Autodesk Inventor part; units mm, degrees
(part 2 of 3)
sketch "Эскиз2" plane through (0, 0, 5) normal (0, 0, 1) x (1, 0, 0)
  circle A0 centre (9.1909, 9.1909) radius 1.6
  line L0 (7.3241, 8.9171) -> (8.619, 7.3929)
  line L1 (8.619, 7.3929) -> (11.0578, 9.4648)
  line L2 (11.0578, 9.4648) -> (9.7628, 10.989)
  line L3 (9.7628, 10.989) -> (7.3241, 8.9171)
  line L4 (7.3241, 8.9171) -> (11.0578, 9.4648) construction
  line L5 (8.619, 7.3929) -> (9.7628, 10.989) construction
  line L6 (7.2492, 10.7043) -> (8.0113, 11.3517)
  line L7 (8.0113, 11.3517) -> (8.9245, 10.2768)
  line L8 (8.9245, 10.2768) -> (8.1624, 9.6293)
  line L9 (8.1624, 9.6293) -> (7.2492, 10.7043)
  circle A1 centre (9.1909, 9.1909) radius 0.5
  line L10 (8.5848, 2.046) -> (8.6119, 2.08)
  line L11 (8.6119, 2.08) -> (8.6454, 2.1135)
  line L12 (8.6454, 2.1135) -> (8.6907, 2.1463)
  line L13 (8.6907, 2.1463) -> (8.8034, 2.1753)
  line L14 (8.8034, 2.1753) -> (9.3579, 2.1666)
  line L15 (9.3579, 2.1666) -> (9.4696, 2.1341)
  line L16 (9.4696, 2.1341) -> (9.5139, 2.0998)
  line L17 (9.5139, 2.0998) -> (9.5464, 2.0653)
  line L18 (9.5464, 2.0653) -> (9.5724, 2.0305)
  line L19 (9.5724, 2.0305) -> (9.5941, 1.9955)
  line L20 (9.5941, 1.9955) -> (9.6287, 1.9253)
  line L21 (9.6287, 1.9253) -> (9.6547, 1.8546)
  line L22 (9.6547, 1.8546) -> (9.6746, 1.7836)
  line L23 (9.6746, 1.7836) -> (9.6894, 1.7122)
  line L24 (9.6894, 1.7122) -> (9.7076, 1.5688)
  line L25 (9.7076, 1.5688) -> (9.7394, 1.4264)
  line L26 (9.7394, 1.4264) -> (9.7859, 1.2851)
  line L27 (9.7859, 1.2851) -> (9.8431, 1.1448)
  line L28 (9.8431, 1.1448) -> (9.9095, 1.0056)
  line L29 (9.9095, 1.0056) -> (9.9841, 0.8675)
  line L30 (9.9841, 0.8675) -> (10.0665, 0.7307)
  line L31 (10.0665, 0.7307) -> (10.1561, 0.5952)
  line L32 (10.1561, 0.5952) -> (10.2527, 0.4612)
  line L33 (10.2527, 0.4612) -> (10.356, 0.3288)
  line L34 (10.356, 0.3288) -> (10.4658, 0.1981)
  line L35 (10.4658, 0.1981) -> (10.5522, 0.1014)
  line L36 (10.5522, 0.1014) -> (11.1304, 0.207)
  line L37 (11.1304, 0.207) -> (11.1771, 0.3281)
  line L38 (11.1771, 0.3281) -> (11.2336, 0.4891)
  line L39 (11.2336, 0.4891) -> (11.2834, 0.6494)
  line L40 (11.2834, 0.6494) -> (11.3264, 0.8089)
  line L41 (11.3264, 0.8089) -> (11.3624, 0.9673)
  line L42 (11.3624, 0.9673) -> (11.3911, 1.1244)
  line L43 (11.3911, 1.1244) -> (11.4121, 1.28)
  line L44 (11.4121, 1.28) -> (11.425, 1.4337)
  line L45 (11.425, 1.4337) -> (11.4289, 1.5851)
  line L46 (11.4289, 1.5851) -> (11.4224, 1.7338)
  line L47 (11.4224, 1.7338) -> (11.4018, 1.8782)
  line L48 (11.4018, 1.8782) -> (11.3682, 2.0188)
  line L49 (11.3682, 2.0188) -> (11.3568, 2.0908)
  line L50 (11.3568, 2.0908) -> (11.3503, 2.1643)
  line L51 (11.3503, 2.1643) -> (11.3497, 2.2396)
  line L52 (11.3497, 2.2396) -> (11.3572, 2.3175)
  line L53 (11.3572, 2.3175) -> (11.3651, 2.3579)
  line L54 (11.3651, 2.3579) -> (11.3772, 2.3996)
  line L55 (11.3772, 2.3996) -> (11.3953, 2.4434)
  line L56 (11.3953, 2.4434) -> (11.4247, 2.4911)
  line L57 (11.4247, 2.4911) -> (11.5177, 2.5611)
  line L58 (11.5177, 2.5611) -> (12.0333, 2.7652)
  line L59 (12.0333, 2.7652) -> (12.149, 2.7779)
  line L60 (12.149, 2.7779) -> (12.203, 2.7632)
  line L61 (12.203, 2.7632) -> (12.2462, 2.7437)
  line L62 (12.2462, 2.7437) -> (12.2835, 2.7215)
  line L63 (12.2835, 2.7215) -> (12.317, 2.6976)
  line L64 (12.317, 2.6976) -> (12.3758, 2.6459)
  line L65 (12.3758, 2.6459) -> (12.4269, 2.5905)
  line L66 (12.4269, 2.5905) -> (12.4724, 2.5325)
  line L67 (12.4724, 2.5325) -> (12.5134, 2.4723)
  line L68 (12.5134, 2.4723) -> (12.5852, 2.3468)
  line L69 (12.5852, 2.3468) -> (12.669, 2.2273)
  line L70 (12.669, 2.2273) -> (12.766, 2.1145)
  line L71 (12.766, 2.1145) -> (12.8726, 2.0068)
  line L72 (12.8726, 2.0068) -> (12.9872, 1.9036)
  line L73 (12.9872, 1.9036) -> (13.109, 1.8046)
  line L74 (13.109, 1.8046) -> (13.2375, 1.7097)
  line L75 (13.2375, 1.7097) -> (13.3721, 1.6189)
  line L76 (13.3721, 1.6189) -> (13.5126, 1.532)
  line L77 (13.5126, 1.532) -> (13.6587, 1.4492)
  line L78 (13.6587, 1.4492) -> (13.8101, 1.3705)
  line L79 (13.8101, 1.3705) -> (13.927, 1.3142)
  line L80 (13.927, 1.3142) -> (14.4208, 1.6331)
  line L81 (14.4208, 1.6331) -> (14.4176, 1.7628)
  line L82 (14.4176, 1.7628) -> (14.4082, 1.9332)
  line L83 (14.4082, 1.9332) -> (14.3928, 2.1004)
  line L84 (14.3928, 2.1004) -> (14.3715, 2.2642)
  line L85 (14.3715, 2.2642) -> (14.3441, 2.4243)
  line L86 (14.3441, 2.4243) -> (14.3105, 2.5804)
  line L87 (14.3105, 2.5804) -> (14.2704, 2.7322)
  line L88 (14.2704, 2.7322) -> (14.2235, 2.8791)
  line L89 (14.2235, 2.8791) -> (14.1692, 3.0205)
  line L90 (14.1692, 3.0205) -> (14.1063, 3.1554)
  line L91 (14.1063, 3.1554) -> (14.032, 3.2809)
  line L92 (14.032, 3.2809) -> (13.9471, 3.398)
  line L93 (13.9471, 3.398) -> (13.9091, 3.4601)
  line L94 (13.9091, 3.4601) -> (13.8749, 3.5255)
  line L95 (13.8749, 3.5255) -> (13.8455, 3.5949)
  line L96 (13.8455, 3.5949) -> (13.8226, 3.6697)
  line L97 (13.8226, 3.6697) -> (13.8145, 3.7101)
  line L98 (13.8145, 3.7101) -> (13.8097, 3.7533)
  line L99 (13.8097, 3.7533) -> (13.8097, 3.8007)
  line L100 (13.8097, 3.8007) -> (13.8185, 3.8559)
  line L101 (13.8185, 3.8559) -> (13.8777, 3.9562)
  line L102 (13.8777, 3.9562) -> (14.2759, 4.3421)
  line L103 (14.2759, 4.3421) -> (14.378, 4.398)
  line L104 (14.378, 4.398) -> (14.4335, 4.4051)
  line L105 (14.4335, 4.4051) -> (14.4809, 4.4036)
  line L106 (14.4809, 4.4036) -> (14.5238, 4.3975)
  line L107 (14.5238, 4.3975) -> (14.5639, 4.3881)
  line L108 (14.5639, 4.3881) -> (14.638, 4.3629)
  line L109 (14.638, 4.3629) -> (14.7065, 4.3313)
  line L110 (14.7065, 4.3313) -> (14.7707, 4.2951)
  line L111 (14.7707, 4.2951) -> (14.8316, 4.2551)
  line L112 (14.8316, 4.2551) -> (14.946, 4.1667)
  line L113 (14.946, 4.1667) -> (15.0691, 4.0884)
  line L114 (15.0691, 4.0884) -> (15.2019, 4.0213)
  line L115 (15.2019, 4.0213) -> (15.3416, 3.9626)
  line L116 (15.3416, 3.9626) -> (15.4869, 3.9111)
  line L117 (15.4869, 3.9111) -> (15.6374, 3.8662)
  line L118 (15.6374, 3.8662) -> (15.7924, 3.8277)
  line L119 (15.7924, 3.8277) -> (15.9515, 3.7953)
  line L120 (15.9515, 3.7953) -> (16.1146, 3.7689)
  line L121 (16.1146, 3.7689) -> (16.2812, 3.7483)
  line L122 (16.2812, 3.7483) -> (16.4512, 3.7335)
  line L123 (16.4512, 3.7335) -> (16.5808, 3.7262)
  line L124 (16.5808, 3.7262) -> (16.915, 4.2097)
  line L125 (16.915, 4.2097) -> (16.8624, 4.3284)
  line L126 (16.8624, 4.3284) -> (16.7885, 4.4822)
  line L127 (16.7885, 4.4822) -> (16.7103, 4.6308)
  line L128 (16.7103, 4.6308) -> (16.6279, 4.774)
  line L129 (16.6279, 4.774) -> (16.5413, 4.9114)
  line L130 (16.5413, 4.9114) -> (16.4505, 5.0428)
  line L131 (16.4505, 5.0428) -> (16.3554, 5.1677)
  line L132 (16.3554, 5.1677) -> (16.2558, 5.2855)
  line L133 (16.2558, 5.2855) -> (16.1515, 5.3953)
  line L134 (16.1515, 5.3953) -> (16.0419, 5.4958)
  line L135 (16.0419, 5.4958) -> (15.9251, 5.5834)
  line L136 (15.9251, 5.5834) -> (15.8019, 5.6591)
  line L137 (15.8019, 5.6591) -> (15.743, 5.7019)
  line L138 (15.743, 5.7019) -> (15.6864, 5.7492)
  line L139 (15.6864, 5.7492) -> (15.6327, 5.8021)
  line L140 (15.6327, 5.8021) -> (15.5829, 5.8625)
  line L141 (15.5829, 5.8625) -> (15.56, 5.8967)
  line L142 (15.56, 5.8967) -> (15.539, 5.9347)
  line L143 (15.539, 5.9347) -> (15.5209, 5.9785)
  line L144 (15.5209, 5.9785) -> (15.5079, 6.0329)
  line L145 (15.5079, 6.0329) -> (15.5242, 6.1482)
  line L146 (15.5242, 6.1482) -> (15.7444, 6.6571)
  line L147 (15.7444, 6.6571) -> (15.8173, 6.7479)
  line L148 (15.8173, 6.7479) -> (15.8658, 6.7757)
  line L149 (15.8658, 6.7757) -> (15.9102, 6.7924)
  line L150 (15.9102, 6.7924) -> (15.9523, 6.8032)
  line L151 (15.9523, 6.8032) -> (15.9929, 6.8099)
  line L152 (15.9929, 6.8099) -> (16.071, 6.8149)
  line L153 (16.071, 6.8149) -> (16.1463, 6.812)
  line L154 (16.1463, 6.812) -> (16.2195, 6.8031)
  line L155 (16.2195, 6.8031) -> (16.2911, 6.7895)
  line L156 (16.2911, 6.7895) -> (16.4306, 6.7515)
  line L157 (16.4306, 6.7515) -> (16.5743, 6.7263)
  line L158 (16.5743, 6.7263) -> (16.7227, 6.7151)
  line L159 (16.7227, 6.7151) -> (16.8742, 6.7143)
  line L160 (16.8742, 6.7143) -> (17.0282, 6.7224)
  line L161 (17.0282, 6.7224) -> (17.1843, 6.7385)
  line L162 (17.1843, 6.7385) -> (17.3423, 6.7622)
  line L163 (17.3423, 6.7622) -> (17.5017, 6.7932)
  line L164 (17.5017, 6.7932) -> (17.6625, 6.8312)
  line L165 (17.6625, 6.8312) -> (17.8243, 6.8759)
  line L166 (17.8243, 6.8759) -> (17.987, 6.9273)
  line L167 (17.987, 6.9273) -> (18.1095, 6.9702)
  line L168 (18.1095, 6.9702) -> (18.2332, 7.5448)
  line L169 (18.2332, 7.5448) -> (18.1392, 7.6343)
  line L170 (18.1392, 7.6343) -> (18.0121, 7.7481)
  line L171 (18.0121, 7.7481) -> (17.883, 7.8555)
  line L172 (17.883, 7.8555) -> (17.7521, 7.9562)
  line L173 (17.7521, 7.9562) -> (17.6195, 8.0501)
  line L174 (17.6195, 8.0501) -> (17.4854, 8.1367)
  line L175 (17.4854, 8.1367) -> (17.3497, 8.2156)
  line L176 (17.3497, 8.2156) -> (17.2126, 8.2864)
  line L177 (17.2126, 8.2864) -> (17.0742, 8.348)
  line L178 (17.0742, 8.348) -> (16.9344, 8.3988)
  line L179 (16.9344, 8.3988) -> (16.7931, 8.4351)
  line L180 (16.7931, 8.4351) -> (16.6503, 8.4578)
  line L181 (16.6503, 8.4578) -> (16.5795, 8.4749)
  line L182 (16.5795, 8.4749) -> (16.5091, 8.4969)
  line L183 (16.5091, 8.4969) -> (16.4393, 8.5252)
  line L184 (16.4393, 8.5252) -> (16.3701, 8.5619)
  line L185 (16.3701, 8.5619) -> (16.3359, 8.5848)
  line L186 (16.3359, 8.5848) -> (16.3019, 8.6119)
  line L187 (16.3019, 8.6119) -> (16.2684, 8.6454)
  line L188 (16.2684, 8.6454) -> (16.2356, 8.6907)
  line L189 (16.2356, 8.6907) -> (16.2065, 8.8034)
  line L190 (16.2065, 8.8034) -> (16.2152, 9.3579)
  line L191 (16.2152, 9.3579) -> (16.2478, 9.4696)
  line L192 (16.2478, 9.4696) -> (16.282, 9.5139)
  line L193 (16.282, 9.5139) -> (16.3166, 9.5464)
  line L194 (16.3166, 9.5464) -> (16.3514, 9.5724)
  line L195 (16.3514, 9.5724) -> (16.3863, 9.5941)
  line L196 (16.3863, 9.5941) -> (16.4566, 9.6287)
  line L197 (16.4566, 9.6287) -> (16.5273, 9.6547)
  line L198 (16.5273, 9.6547) -> (16.5983, 9.6746)
  line L199 (16.5983, 9.6746) -> (16.6696, 9.6894)
  line L200 (16.6696, 9.6894) -> (16.813, 9.7076)
  line L201 (16.813, 9.7076) -> (16.9555, 9.7394)
  line L202 (16.9555, 9.7394) -> (17.0968, 9.7859)
  line L203 (17.0968, 9.7859) -> (17.2371, 9.8431)
  line L204 (17.2371, 9.8431) -> (17.3763, 9.9095)
  line L205 (17.3763, 9.9095) -> (17.5144, 9.9841)
  line L206 (17.5144, 9.9841) -> (17.6512, 10.0665)
  line L207 (17.6512, 10.0665) -> (17.7867, 10.1561)
  line L208 (17.7867, 10.1561) -> (17.9207, 10.2527)
  line L209 (17.9207, 10.2527) -> (18.0531, 10.356)
  line L210 (18.0531, 10.356) -> (18.1837, 10.4658)
  line L211 (18.1837, 10.4658) -> (18.2805, 10.5522)
  line L212 (18.2805, 10.5522) -> (18.1749, 11.1304)
  line L213 (18.1749, 11.1304) -> (18.0538, 11.1771)
  line L214 (18.0538, 11.1771) -> (17.8928, 11.2336)
  line L215 (17.8928, 11.2336) -> (17.7324, 11.2834)
  line L216 (17.7324, 11.2834) -> (17.5729, 11.3264)
  line L217 (17.5729, 11.3264) -> (17.4145, 11.3624)
  line L218 (17.4145, 11.3624) -> (17.2574, 11.3911)
  line L219 (17.2574, 11.3911) -> (17.1019, 11.4121)
  line L220 (17.1019, 11.4121) -> (16.9482, 11.425)
  line L221 (16.9482, 11.425) -> (16.7967, 11.4289)
  line L222 (16.7967, 11.4289) -> (16.6481, 11.4224)
  line L223 (16.6481, 11.4224) -> (16.5036, 11.4018)
  line L224 (16.5036, 11.4018) -> (16.363, 11.3682)
  line L225 (16.363, 11.3682) -> (16.2911, 11.3568)
  line L226 (16.2911, 11.3568) -> (16.2176, 11.3503)
  line L227 (16.2176, 11.3503) -> (16.1423, 11.3497)
  line L228 (16.1423, 11.3497) -> (16.0643, 11.3572)
  line L229 (16.0643, 11.3572) -> (16.0239, 11.3651)
  line L230 (16.0239, 11.3651) -> (15.9822, 11.3772)
  line L231 (15.9822, 11.3772) -> (15.9384, 11.3953)
  line L232 (15.9384, 11.3953) -> (15.8907, 11.4247)
  line L233 (15.8907, 11.4247) -> (15.8208, 11.5177)
  line L234 (15.8208, 11.5177) -> (15.6166, 12.0333)
  line L235 (15.6166, 12.0333) -> (15.604, 12.149)
  line L236 (15.604, 12.149) -> (15.6187, 12.203)
  line L237 (15.6187, 12.203) -> (15.6382, 12.2462)
  line L238 (15.6382, 12.2462) -> (15.6603, 12.2835)
  line L239 (15.6603, 12.2835) -> (15.6843, 12.317)
  line L240 (15.6843, 12.317) -> (15.736, 12.3758)
  line L241 (15.736, 12.3758) -> (15.7913, 12.4269)
  line L242 (15.7913, 12.4269) -> (15.8494, 12.4724)
  line L243 (15.8494, 12.4724) -> (15.9096, 12.5134)
  line L244 (15.9096, 12.5134) -> (16.0351, 12.5852)
  line L245 (16.0351, 12.5852) -> (16.1546, 12.669)
  line L246 (16.1546, 12.669) -> (16.2673, 12.766)
  line L247 (16.2673, 12.766) -> (16.375, 12.8726)
  line L248 (16.375, 12.8726) -> (16.4783, 12.9872)
  line L249 (16.4783, 12.9872) -> (16.5772, 13.109)
  line L250 (16.5772, 13.109) -> (16.6721, 13.2375)
  line L251 (16.6721, 13.2375) -> (16.763, 13.3721)
  line L252 (16.763, 13.3721) -> (16.8498, 13.5126)
  line L253 (16.8498, 13.5126) -> (16.9326, 13.6587)
  line L254 (16.9326, 13.6587) -> (17.0113, 13.8101)
  line L255 (17.0113, 13.8101) -> (17.0676, 13.927)
  line L256 (17.0676, 13.927) -> (16.7488, 14.4208)
  line L257 (16.7488, 14.4208) -> (16.6191, 14.4176)
  line L258 (16.6191, 14.4176) -> (16.4487, 14.4082)
  line L259 (16.4487, 14.4082) -> (16.2815, 14.3928)
  line L260 (16.2815, 14.3928) -> (16.1177, 14.3715)
  line L261 (16.1177, 14.3715) -> (15.9576, 14.3441)
  line L262 (15.9576, 14.3441) -> (15.8015, 14.3105)
  line L263 (15.8015, 14.3105) -> (15.6497, 14.2704)
  line L264 (15.6497, 14.2704) -> (15.5028, 14.2235)
  line L265 (15.5028, 14.2235) -> (15.3613, 14.1692)
  line L266 (15.3613, 14.1692) -> (15.2265, 14.1063)
  line L267 (15.2265, 14.1063) -> (15.1009, 14.032)
  line L268 (15.1009, 14.032) -> (14.9839, 13.9471)
  line L269 (14.9839, 13.9471) -> (14.9217, 13.9091)
  line L270 (14.9217, 13.9091) -> (14.8564, 13.8749)
  line L271 (14.8564, 13.8749) -> (14.787, 13.8455)
  line L272 (14.787, 13.8455) -> (14.7121, 13.8226)
  line L273 (14.7121, 13.8226) -> (14.6718, 13.8145)
  line L274 (14.6718, 13.8145) -> (14.6286, 13.8097)
  line L275 (14.6286, 13.8097) -> (14.5812, 13.8097)
  line L276 (14.5812, 13.8097) -> (14.5259, 13.8185)
  line L277 (14.5259, 13.8185) -> (14.4257, 13.8777)
  line L278 (14.4257, 13.8777) -> (14.0398, 14.2759)
  line L279 (14.0398, 14.2759) -> (13.9838, 14.378)
  line L280 (13.9838, 14.378) -> (13.9767, 14.4335)
  line L281 (13.9767, 14.4335) -> (13.9782, 14.4809)
  line L282 (13.9782, 14.4809) -> (13.9844, 14.5238)
  line L283 (13.9844, 14.5238) -> (13.9938, 14.5639)
  line L284 (13.9938, 14.5639) -> (14.019, 14.638)
  line L285 (14.019, 14.638) -> (14.0505, 14.7065)
  line L286 (14.0505, 14.7065) -> (14.0868, 14.7707)
  line L287 (14.0868, 14.7707) -> (14.1267, 14.8316)
  line L288 (14.1267, 14.8316) -> (14.2152, 14.946)
  line L289 (14.2152, 14.946) -> (14.2935, 15.0691)
  line L290 (14.2935, 15.0691) -> (14.3605, 15.2019)
  line L291 (14.3605, 15.2019) -> (14.4193, 15.3416)
  line L292 (14.4193, 15.3416) -> (14.4708, 15.4869)
  line L293 (14.4708, 15.4869) -> (14.5156, 15.6374)
  line L294 (14.5156, 15.6374) -> (14.5541, 15.7924)
  line L295 (14.5541, 15.7924) -> (14.5866, 15.9515)
  line L296 (14.5866, 15.9515) -> (14.613, 16.1146)
  line L297 (14.613, 16.1146) -> (14.6336, 16.2812)
  line L298 (14.6336, 16.2812) -> (14.6484, 16.4512)
  line L299 (14.6484, 16.4512) -> (14.6556, 16.5808)
  line L300 (14.6556, 16.5808) -> (14.1721, 16.915)
  line L301 (14.1721, 16.915) -> (14.0535, 16.8624)
  line L302 (14.0535, 16.8624) -> (13.8997, 16.7885)
  line L303 (13.8997, 16.7885) -> (13.7511, 16.7103)
  line L304 (13.7511, 16.7103) -> (13.6079, 16.6279)
  line L305 (13.6079, 16.6279) -> (13.4704, 16.5413)
  line L306 (13.4704, 16.5413) -> (13.3391, 16.4505)
  line L307 (13.3391, 16.4505) -> (13.2142, 16.3554)
  line L308 (13.2142, 16.3554) -> (13.0964, 16.2558)
  line L309 (13.0964, 16.2558) -> (12.9865, 16.1515)
  line L310 (12.9865, 16.1515) -> (12.886, 16.0419)
  line L311 (12.886, 16.0419) -> (12.7985, 15.9251)
  line L312 (12.7985, 15.9251) -> (12.7228, 15.8019)
  line L313 (12.7228, 15.8019) -> (12.6799, 15.743)
  line L314 (12.6799, 15.743) -> (12.6327, 15.6864)
  line L315 (12.6327, 15.6864) -> (12.5798, 15.6327)
  line L316 (12.5798, 15.6327) -> (12.5194, 15.5829)
  line L317 (12.5194, 15.5829) -> (12.4852, 15.56)
  line L318 (12.4852, 15.56) -> (12.4472, 15.539)
  line L319 (12.4472, 15.539) -> (12.4034, 15.5209)
  line L320 (12.4034, 15.5209) -> (12.3489, 15.5079)
  line L321 (12.3489, 15.5079) -> (12.2337, 15.5242)
  line L322 (12.2337, 15.5242) -> (11.7248, 15.7444)
  line L323 (11.7248, 15.7444) -> (11.634, 15.8173)
  line L324 (11.634, 15.8173) -> (11.6062, 15.8658)
  line L325 (11.6062, 15.8658) -> (11.5894, 15.9102)
  line L326 (11.5894, 15.9102) -> (11.5787, 15.9523)
  line L327 (11.5787, 15.9523) -> (11.572, 15.9929)
  line L328 (11.572, 15.9929) -> (11.567, 16.071)
  line L329 (11.567, 16.071) -> (11.5699, 16.1463)
  line L330 (11.5699, 16.1463) -> (11.5788, 16.2195)
  line L331 (11.5788, 16.2195) -> (11.5924, 16.2911)
  line L332 (11.5924, 16.2911) -> (11.6304, 16.4306)
  line L333 (11.6304, 16.4306) -> (11.6556, 16.5743)
  line L334 (11.6556, 16.5743) -> (11.6667, 16.7227)
  line L335 (11.6667, 16.7227) -> (11.6676, 16.8742)
  line L336 (11.6676, 16.8742) -> (11.6595, 17.0282)
  line L337 (11.6595, 17.0282) -> (11.6434, 17.1843)
  line L338 (11.6434, 17.1843) -> (11.6196, 17.3423)
  line L339 (11.6196, 17.3423) -> (11.5887, 17.5017)
  line L340 (11.5887, 17.5017) -> (11.5507, 17.6625)
  line L341 (11.5507, 17.6625) -> (11.506, 17.8243)
  line L342 (11.506, 17.8243) -> (11.4545, 17.987)
  line L343 (11.4545, 17.987) -> (11.4117, 18.1095)
  line L344 (11.4117, 18.1095) -> (10.8371, 18.2332)
  line L345 (10.8371, 18.2332) -> (10.7476, 18.1392)
  line L346 (10.7476, 18.1392) -> (10.6338, 18.0121)
  line L347 (10.6338, 18.0121) -> (10.5264, 17.883)
  line L348 (10.5264, 17.883) -> (10.4256, 17.7521)
  line L349 (10.4256, 17.7521) -> (10.3318, 17.6195)
  line L350 (10.3318, 17.6195) -> (10.2452, 17.4854)
  line L351 (10.2452, 17.4854) -> (10.1662, 17.3497)
  line L352 (10.1662, 17.3497) -> (10.0955, 17.2126)
  line L353 (10.0955, 17.2126) -> (10.0339, 17.0742)
  line L354 (10.0339, 17.0742) -> (9.983, 16.9344)
  line L355 (9.983, 16.9344) -> (9.9468, 16.7931)
  line L356 (9.9468, 16.7931) -> (9.924, 16.6503)
  line L357 (9.924, 16.6503) -> (9.907, 16.5795)
  line L358 (9.907, 16.5795) -> (9.885, 16.5091)
  line L359 (9.885, 16.5091) -> (9.8567, 16.4393)
  line L360 (9.8567, 16.4393) -> (9.8199, 16.3701)
  line L361 (9.8199, 16.3701) -> (9.7971, 16.3359)
  line L362 (9.7971, 16.3359) -> (9.77, 16.3019)
  line L363 (9.77, 16.3019) -> (9.7365, 16.2684)
  line L364 (9.7365, 16.2684) -> (9.6911, 16.2356)
  line L365 (9.6911, 16.2356) -> (9.5784, 16.2065)
  line L366 (9.5784, 16.2065) -> (9.024, 16.2152)
  line L367 (9.024, 16.2152) -> (8.9122, 16.2478)
  line L368 (8.9122, 16.2478) -> (8.868, 16.282)
  line L369 (8.868, 16.282) -> (8.8355, 16.3166)
  line L370 (8.8355, 16.3166) -> (8.8095, 16.3514)
  line L371 (8.8095, 16.3514) -> (8.7878, 16.3863)
  line L372 (8.7878, 16.3863) -> (8.7532, 16.4566)
  line L373 (8.7532, 16.4566) -> (8.7271, 16.5273)
  line L374 (8.7271, 16.5273) -> (8.7073, 16.5983)
  line L375 (8.7073, 16.5983) -> (8.6925, 16.6696)
  line L376 (8.6925, 16.6696) -> (8.6742, 16.813)
  line L377 (8.6742, 16.813) -> (8.6425, 16.9555)
  line L378 (8.6425, 16.9555) -> (8.596, 17.0968)
  line L379 (8.596, 17.0968) -> (8.5388, 17.2371)
  line L380 (8.5388, 17.2371) -> (8.4724, 17.3763)
  line L381 (8.4724, 17.3763) -> (8.3977, 17.5144)
  line L382 (8.3977, 17.5144) -> (8.3154, 17.6512)
  line L383 (8.3154, 17.6512) -> (8.2257, 17.7867)
  line L384 (8.2257, 17.7867) -> (8.1291, 17.9207)
  line L385 (8.1291, 17.9207) -> (8.0259, 18.0531)
  line L386 (8.0259, 18.0531) -> (7.9161, 18.1837)
  line L387 (7.9161, 18.1837) -> (7.8296, 18.2805)
  line L388 (7.8296, 18.2805) -> (7.2514, 18.1749)
  line L389 (7.2514, 18.1749) -> (7.2047, 18.0538)
  line L390 (7.2047, 18.0538) -> (7.1482, 17.8928)
  line L391 (7.1482, 17.8928) -> (7.0984, 17.7324)
  line L392 (7.0984, 17.7324) -> (7.0554, 17.5729)
  line L393 (7.0554, 17.5729) -> (7.0195, 17.4145)
  line L394 (7.0195, 17.4145) -> (6.9908, 17.2574)
  line L395 (6.9908, 17.2574) -> (6.9698, 17.1019)
  line L396 (6.9698, 17.1019) -> (6.9569, 16.9482)
  line L397 (6.9569, 16.9482) -> (6.9529, 16.7967)
  line L398 (6.9529, 16.7967) -> (6.9594, 16.6481)
  line L399 (6.9594, 16.6481) -> (6.9801, 16.5036)
  line L400 (6.9801, 16.5036) -> (7.0137, 16.363)
  line L401 (7.0137, 16.363) -> (7.025, 16.2911)
  line L402 (7.025, 16.2911) -> (7.0316, 16.2176)
  line L403 (7.0316, 16.2176) -> (7.0322, 16.1423)
  line L404 (7.0322, 16.1423) -> (7.0247, 16.0643)
  line L405 (7.0247, 16.0643) -> (7.0167, 16.0239)
  line L406 (7.0167, 16.0239) -> (7.0047, 15.9822)
  line L407 (7.0047, 15.9822) -> (6.9865, 15.9384)
  line L408 (6.9865, 15.9384) -> (6.9572, 15.8907)
  line L409 (6.9572, 15.8907) -> (6.8642, 15.8208)
  line L410 (6.8642, 15.8208) -> (6.3486, 15.6166)
  line L411 (6.3486, 15.6166) -> (6.2329, 15.604)
  line L412 (6.2329, 15.604) -> (6.1789, 15.6187)
  line L413 (6.1789, 15.6187) -> (6.1357, 15.6382)
  line L414 (6.1357, 15.6382) -> (6.0983, 15.6603)
  line L415 (6.0983, 15.6603) -> (6.0649, 15.6843)
  line L416 (6.0649, 15.6843) -> (6.0061, 15.736)
  line L417 (6.0061, 15.736) -> (5.9549, 15.7913)
  line L418 (5.9549, 15.7913) -> (5.9094, 15.8494)
  line L419 (5.9094, 15.8494) -> (5.8685, 15.9096)
  line L420 (5.8685, 15.9096) -> (5.7967, 16.0351)
  line L421 (5.7967, 16.0351) -> (5.7129, 16.1546)
  line L422 (5.7129, 16.1546) -> (5.6158, 16.2673)
  line L423 (5.6158, 16.2673) -> (5.5093, 16.375)
  line L424 (5.5093, 16.375) -> (5.3947, 16.4783)
  line L425 (5.3947, 16.4783) -> (5.2729, 16.5772)
  line L426 (5.2729, 16.5772) -> (5.1444, 16.6721)
  line L427 (5.1444, 16.6721) -> (5.0098, 16.763)
  line L428 (5.0098, 16.763) -> (4.8692, 16.8498)
  line L429 (4.8692, 16.8498) -> (4.7232, 16.9326)
  line L430 (4.7232, 16.9326) -> (4.5717, 17.0113)
  line L431 (4.5717, 17.0113) -> (4.4548, 17.0676)
  line L432 (4.4548, 17.0676) -> (3.961, 16.7488)
  line L433 (3.961, 16.7488) -> (3.9643, 16.6191)
  line L434 (3.9643, 16.6191) -> (3.9737, 16.4487)
  line L435 (3.9737, 16.4487) -> (3.989, 16.2815)
  line L436 (3.989, 16.2815) -> (4.0103, 16.1177)
  line L437 (4.0103, 16.1177) -> (4.0377, 15.9576)
  line L438 (4.0377, 15.9576) -> (4.0714, 15.8015)
  line L439 (4.0714, 15.8015) -> (4.1115, 15.6497)
  line L440 (4.1115, 15.6497) -> (4.1584, 15.5028)
  line L441 (4.1584, 15.5028) -> (4.2127, 15.3613)
  line L442 (4.2127, 15.3613) -> (4.2755, 15.2265)
  line L443 (4.2755, 15.2265) -> (4.3499, 15.1009)
  line L444 (4.3499, 15.1009) -> (4.4348, 14.9839)
  line L445 (4.4348, 14.9839) -> (4.4728, 14.9217)
  line L446 (4.4728, 14.9217) -> (4.507, 14.8564)
  line L447 (4.507, 14.8564) -> (4.5364, 14.787)
  line L448 (4.5364, 14.787) -> (4.5593, 14.7121)
  line L449 (4.5593, 14.7121) -> (4.5673, 14.6718)
  line L450 (4.5673, 14.6718) -> (4.5722, 14.6286)
  line L451 (4.5722, 14.6286) -> (4.5722, 14.5812)
  line L452 (4.5722, 14.5812) -> (4.5633, 14.5259)
  line L453 (4.5633, 14.5259) -> (4.5042, 14.4257)
  line L454 (4.5042, 14.4257) -> (4.106, 14.0398)
  line L455 (4.106, 14.0398) -> (4.0039, 13.9838)
  line L456 (4.0039, 13.9838) -> (3.9484, 13.9767)
  line L457 (3.9484, 13.9767) -> (3.901, 13.9782)
  line L458 (3.901, 13.9782) -> (3.858, 13.9844)
  line L459 (3.858, 13.9844) -> (3.8179, 13.9938)
  line L460 (3.8179, 13.9938) -> (3.7438, 14.019)
  line L461 (3.7438, 14.019) -> (3.6754, 14.0505)
  line L462 (3.6754, 14.0505) -> (3.6112, 14.0868)
  line L463 (3.6112, 14.0868) -> (3.5502, 14.1267)
  line L464 (3.5502, 14.1267) -> (3.4359, 14.2152)
  line L465 (3.4359, 14.2152) -> (3.3127, 14.2935)
  line L466 (3.3127, 14.2935) -> (3.18, 14.3605)
  line L467 (3.18, 14.3605) -> (3.0403, 14.4193)
  line L468 (3.0403, 14.4193) -> (2.8949, 14.4708)
  line L469 (2.8949, 14.4708) -> (2.7445, 14.5156)
  line L470 (2.7445, 14.5156) -> (2.5895, 14.5541)
  line L471 (2.5895, 14.5541) -> (2.4303, 14.5866)
  line L472 (2.4303, 14.5866) -> (2.2673, 14.613)
  line L473 (2.2673, 14.613) -> (2.1006, 14.6336)
  line L474 (2.1006, 14.6336) -> (1.9306, 14.6484)
  line L475 (1.9306, 14.6484) -> (1.8011, 14.6556)
  line L476 (1.8011, 14.6556) -> (1.4669, 14.1721)
  line L477 (1.4669, 14.1721) -> (1.5195, 14.0535)
  line L478 (1.5195, 14.0535) -> (1.5934, 13.8997)
  line L479 (1.5934, 13.8997) -> (1.6716, 13.7511)
  line L480 (1.6716, 13.7511) -> (1.7539, 13.6079)
  line L481 (1.7539, 13.6079) -> (1.8405, 13.4704)
  line L482 (1.8405, 13.4704) -> (1.9313, 13.3391)
  line L483 (1.9313, 13.3391) -> (2.0265, 13.2142)
  line L484 (2.0265, 13.2142) -> (2.126, 13.0964)
  line L485 (2.126, 13.0964) -> (2.2303, 12.9865)
  line L486 (2.2303, 12.9865) -> (2.34, 12.886)
  line L487 (2.34, 12.886) -> (2.4568, 12.7985)
  line L488 (2.4568, 12.7985) -> (2.5799, 12.7228)
  line L489 (2.5799, 12.7228) -> (2.6389, 12.6799)
  line L490 (2.6389, 12.6799) -> (2.6954, 12.6327)
  line L491 (2.6954, 12.6327) -> (2.7491, 12.5798)
  line L492 (2.7491, 12.5798) -> (2.799, 12.5194)
  line L493 (2.799, 12.5194) -> (2.8219, 12.4852)
  line L494 (2.8219, 12.4852) -> (2.8428, 12.4472)
  line L495 (2.8428, 12.4472) -> (2.861, 12.4034)
  line L496 (2.861, 12.4034) -> (2.874, 12.3489)
  line L497 (2.874, 12.3489) -> (2.8577, 12.2337)
  line L498 (2.8577, 12.2337) -> (2.6374, 11.7248)
  line L499 (2.6374, 11.7248) -> (2.5646, 11.634)
  line L500 (2.5646, 11.634) -> (2.516, 11.6062)
  line L501 (2.516, 11.6062) -> (2.4717, 11.5894)
  line L502 (2.4717, 11.5894) -> (2.4296, 11.5787)
  line L503 (2.4296, 11.5787) -> (2.389, 11.572)
  line L504 (2.389, 11.572) -> (2.3108, 11.567)
  line L505 (2.3108, 11.567) -> (2.2356, 11.5699)
  line L506 (2.2356, 11.5699) -> (2.1623, 11.5788)
  line L507 (2.1623, 11.5788) -> (2.0908, 11.5924)
  line L508 (2.0908, 11.5924) -> (1.9513, 11.6304)
  line L509 (1.9513, 11.6304) -> (1.8075, 11.6556)
  line L510 (1.8075, 11.6556) -> (1.6592, 11.6667)
  line L511 (1.6592, 11.6667) -> (1.5077, 11.6676)
  line L512 (1.5077, 11.6676) -> (1.3537, 11.6595)
  line L513 (1.3537, 11.6595) -> (1.1975, 11.6434)
  line L514 (1.1975, 11.6434) -> (1.0396, 11.6196)
  line L515 (1.0396, 11.6196) -> (0.8801, 11.5887)
  line L516 (0.8801, 11.5887) -> (0.7194, 11.5507)
  line L517 (0.7194, 11.5507) -> (0.5575, 11.506)
  line L518 (0.5575, 11.506) -> (0.3948, 11.4545)
  line L519 (0.3948, 11.4545) -> (0.2723, 11.4117)
  line L520 (0.2723, 11.4117) -> (0.1486, 10.8371)
  line L521 (0.1486, 10.8371) -> (0.2426, 10.7476)
  line L522 (0.2426, 10.7476) -> (0.3698, 10.6338)
  line L523 (0.3698, 10.6338) -> (0.4988, 10.5264)
  line L524 (0.4988, 10.5264) -> (0.6297, 10.4256)
  line L525 (0.6297, 10.4256) -> (0.7623, 10.3318)
  line L526 (0.7623, 10.3318) -> (0.8965, 10.2452)
  line L527 (0.8965, 10.2452) -> (1.0322, 10.1662)
  line L528 (1.0322, 10.1662) -> (1.1692, 10.0955)
  line L529 (1.1692, 10.0955) -> (1.3077, 10.0339)
  line L530 (1.3077, 10.0339) -> (1.4474, 9.983)
  line L531 (1.4474, 9.983) -> (1.5888, 9.9468)
  line L532 (1.5888, 9.9468) -> (1.7316, 9.924)
  line L533 (1.7316, 9.924) -> (1.8024, 9.907)
  line L534 (1.8024, 9.907) -> (1.8728, 9.885)
  line L535 (1.8728, 9.885) -> (1.9426, 9.8567)
  line L536 (1.9426, 9.8567) -> (2.0118, 9.8199)
  line L537 (2.0118, 9.8199) -> (2.046, 9.7971)
  line L538 (2.046, 9.7971) -> (2.08, 9.77)
  line L539 (2.08, 9.77) -> (2.1135, 9.7365)
  line L540 (2.1135, 9.7365) -> (2.1463, 9.6911)
  line L541 (2.1463, 9.6911) -> (2.1753, 9.5784)
  line L542 (2.1753, 9.5784) -> (2.1666, 9.024)
  line L543 (2.1666, 9.024) -> (2.1341, 8.9122)
  line L544 (2.1341, 8.9122) -> (2.0998, 8.868)
  line L545 (2.0998, 8.868) -> (2.0653, 8.8355)
  line L546 (2.0653, 8.8355) -> (2.0305, 8.8095)
  line L547 (2.0305, 8.8095) -> (1.9956, 8.7878)
  line L548 (1.9956, 8.7878) -> (1.9253, 8.7532)
  line L549 (1.9253, 8.7532) -> (1.8546, 8.7271)
  line L550 (1.8546, 8.7271) -> (1.7836, 8.7073)
  line L551 (1.7836, 8.7073) -> (1.7122, 8.6925)
  line L552 (1.7122, 8.6925) -> (1.5688, 8.6742)
  line L553 (1.5688, 8.6742) -> (1.4264, 8.6425)
  line L554 (1.4264, 8.6425) -> (1.2851, 8.596)
  line L555 (1.2851, 8.596) -> (1.1448, 8.5388)
  line L556 (1.1448, 8.5388) -> (1.0056, 8.4724)
  line L557 (1.0056, 8.4724) -> (0.8675, 8.3977)
  line L558 (0.8675, 8.3977) -> (0.7307, 8.3154)
  line L559 (0.7307, 8.3154) -> (0.5952, 8.2257)
  line L560 (0.5952, 8.2257) -> (0.4612, 8.1291)
  line L561 (0.4612, 8.1291) -> (0.3288, 8.0259)
  line L562 (0.3288, 8.0259) -> (0.1981, 7.9161)
  line L563 (0.1981, 7.9161) -> (0.1014, 7.8296)
  line L564 (0.1014, 7.8296) -> (0.207, 7.2514)
  line L565 (0.207, 7.2514) -> (0.3281, 7.2047)
  line L566 (0.3281, 7.2047) -> (0.4891, 7.1482)
  line L567 (0.4891, 7.1482) -> (0.6494, 7.0984)
  line L568 (0.6494, 7.0984) -> (0.8089, 7.0554)
  line L569 (0.8089, 7.0554) -> (0.9673, 7.0195)
  line L570 (0.9673, 7.0195) -> (1.1244, 6.9908)
  line L571 (1.1244, 6.9908) -> (1.28, 6.9698)
  line L572 (1.28, 6.9698) -> (1.4337, 6.9569)
  line L573 (1.4337, 6.9569) -> (1.5851, 6.9529)
  line L574 (1.5851, 6.9529) -> (1.7337, 6.9594)
  line L575 (1.7337, 6.9594) -> (1.8782, 6.9801)
  line L576 (1.8782, 6.9801) -> (2.0188, 7.0137)
  line L577 (2.0188, 7.0137) -> (2.0908, 7.025)
  line L578 (2.0908, 7.025) -> (2.1643, 7.0316)
  line L579 (2.1643, 7.0316) -> (2.2396, 7.0322)
  line L580 (2.2396, 7.0322) -> (2.3175, 7.0247)
  line L581 (2.3175, 7.0247) -> (2.3579, 7.0167)
  line L582 (2.3579, 7.0167) -> (2.3996, 7.0047)
  line L583 (2.3996, 7.0047) -> (2.4435, 6.9865)
  line L584 (2.4435, 6.9865) -> (2.4911, 6.9572)
  line L585 (2.4911, 6.9572) -> (2.5611, 6.8642)
  line L586 (2.5611, 6.8642) -> (2.7652, 6.3486)
  line L587 (2.7652, 6.3486) -> (2.7779, 6.2329)
  line L588 (2.7779, 6.2329) -> (2.7632, 6.1789)
  line L589 (2.7632, 6.1789) -> (2.7437, 6.1357)
  line L590 (2.7437, 6.1357) -> (2.7215, 6.0983)
  line L591 (2.7215, 6.0983) -> (2.6976, 6.0649)
  line L592 (2.6976, 6.0649) -> (2.6459, 6.0061)
  line L593 (2.6459, 6.0061) -> (2.5905, 5.9549)
  line L594 (2.5905, 5.9549) -> (2.5325, 5.9094)
  line L595 (2.5325, 5.9094) -> (2.4723, 5.8685)
  line L596 (2.4723, 5.8685) -> (2.3468, 5.7967)
  line L597 (2.3468, 5.7967) -> (2.2273, 5.7129)
  line L598 (2.2273, 5.7129) -> (2.1145, 5.6158)
  line L599 (2.1145, 5.6158) -> (2.0068, 5.5093)
  line L600 (2.0068, 5.5093) -> (1.9036, 5.3947)
  line L601 (1.9036, 5.3947) -> (1.8046, 5.2729)
  line L602 (1.8046, 5.2729) -> (1.7097, 5.1444)
  line L603 (1.7097, 5.1444) -> (1.6189, 5.0098)
  line L604 (1.6189, 5.0098) -> (1.532, 4.8692)
  line L605 (1.532, 4.8692) -> (1.4492, 4.7232)
  line L606 (1.4492, 4.7232) -> (1.3705, 4.5717)
  line L607 (1.3705, 4.5717) -> (1.3142, 4.4548)
  line L608 (1.3142, 4.4548) -> (1.6331, 3.961)
  line L609 (1.6331, 3.961) -> (1.7628, 3.9643)
  line L610 (1.7628, 3.9643) -> (1.9332, 3.9737)
  line L611 (1.9332, 3.9737) -> (2.1004, 3.989)
  line L612 (2.1004, 3.989) -> (2.2642, 4.0103)
  line L613 (2.2642, 4.0103) -> (2.4243, 4.0377)
  line L614 (2.4243, 4.0377) -> (2.5804, 4.0714)
  line L615 (2.5804, 4.0714) -> (2.7322, 4.1115)
  line L616 (2.7322, 4.1115) -> (2.8791, 4.1584)
  line L617 (2.8791, 4.1584) -> (3.0205, 4.2127)
  line L618 (3.0205, 4.2127) -> (3.1554, 4.2755)
  line L619 (3.1554, 4.2755) -> (3.2809, 4.3499)
  line L620 (3.2809, 4.3499) -> (3.398, 4.4348)
  line L621 (3.398, 4.4348) -> (3.4601, 4.4728)
  line L622 (3.4601, 4.4728) -> (3.5255, 4.507)
  line L623 (3.5255, 4.507) -> (3.5949, 4.5364)
  line L624 (3.5949, 4.5364) -> (3.6697, 4.5593)
  line L625 (3.6697, 4.5593) -> (3.7101, 4.5673)
  line L626 (3.7101, 4.5673) -> (3.7533, 4.5722)
  line L627 (3.7533, 4.5722) -> (3.8007, 4.5722)
  line L628 (3.8007, 4.5722) -> (3.8559, 4.5633)
  line L629 (3.8559, 4.5633) -> (3.9562, 4.5042)
  line L630 (3.9562, 4.5042) -> (4.3421, 4.106)
  line L631 (4.3421, 4.106) -> (4.398, 4.0039)
  line L632 (4.398, 4.0039) -> (4.4051, 3.9484)
  line L633 (4.4051, 3.9484) -> (4.4036, 3.901)
  line L634 (4.4036, 3.901) -> (4.3975, 3.858)
  line L635 (4.3975, 3.858) -> (4.3881, 3.8179)
  line L636 (4.3881, 3.8179) -> (4.3629, 3.7438)
  line L637 (4.3629, 3.7438) -> (4.3313, 3.6754)
  line L638 (4.3313, 3.6754) -> (4.2951, 3.6112)
  line L639 (4.2951, 3.6112) -> (4.2551, 3.5502)
  line L640 (4.2551, 3.5502) -> (4.1667, 3.4359)
  line L641 (4.1667, 3.4359) -> (4.0884, 3.3127)
  line L642 (4.0884, 3.3127) -> (4.0213, 3.18)
  line L643 (4.0213, 3.18) -> (3.9626, 3.0403)
  line L644 (3.9626, 3.0403) -> (3.9111, 2.8949)
  line L645 (3.9111, 2.8949) -> (3.8662, 2.7445)
  line L646 (3.8662, 2.7445) -> (3.8277, 2.5895)
  line L647 (3.8277, 2.5895) -> (3.7953, 2.4303)
  line L648 (3.7953, 2.4303) -> (3.7689, 2.2673)
  line L649 (3.7689, 2.2673) -> (3.7483, 2.1006)
  line L650 (3.7483, 2.1006) -> (3.7335, 1.9306)
  line L651 (3.7335, 1.9306) -> (3.7262, 1.8011)
  line L652 (3.7262, 1.8011) -> (4.2097, 1.4669)
  line L653 (4.2097, 1.4669) -> (4.3284, 1.5195)
  line L654 (4.3284, 1.5195) -> (4.4822, 1.5934)
  line L655 (4.4822, 1.5934) -> (4.6308, 1.6716)
  line L656 (4.6308, 1.6716) -> (4.774, 1.7539)
  line L657 (4.774, 1.7539) -> (4.9114, 1.8405)
  line L658 (4.9114, 1.8405) -> (5.0428, 1.9313)
  line L659 (5.0428, 1.9313) -> (5.1677, 2.0265)
  line L660 (5.1677, 2.0265) -> (5.2855, 2.126)
  line L661 (5.2855, 2.126) -> (5.3953, 2.2303)
  line L662 (5.3953, 2.2303) -> (5.4958, 2.34)
  line L663 (5.4958, 2.34) -> (5.5834, 2.4568)
  line L664 (5.5834, 2.4568) -> (5.6591, 2.5799)
  line L665 (5.6591, 2.5799) -> (5.7019, 2.6389)
  line L666 (5.7019, 2.6389) -> (5.7492, 2.6954)
  line L667 (5.7492, 2.6954) -> (5.8021, 2.7491)
  line L668 (5.8021, 2.7491) -> (5.8625, 2.799)
  line L669 (5.8625, 2.799) -> (5.8967, 2.8219)
  line L670 (5.8967, 2.8219) -> (5.9347, 2.8428)
  line L671 (5.9347, 2.8428) -> (5.9785, 2.861)
  line L672 (5.9785, 2.861) -> (6.0329, 2.874)
  line L673 (6.0329, 2.874) -> (6.1482, 2.8577)
  line L674 (6.1482, 2.8577) -> (6.6571, 2.6374)
  line L675 (6.6571, 2.6374) -> (6.7479, 2.5646)
  line L676 (6.7479, 2.5646) -> (6.7757, 2.516)
  line L677 (6.7757, 2.516) -> (6.7924, 2.4717)
  line L678 (6.7924, 2.4717) -> (6.8032, 2.4296)
  line L679 (6.8032, 2.4296) -> (6.8099, 2.389)
  line L680 (6.8099, 2.389) -> (6.8149, 2.3108)
  line L681 (6.8149, 2.3108) -> (6.812, 2.2355)
  line L682 (6.812, 2.2355) -> (6.8031, 2.1623)
  line L683 (6.8031, 2.1623) -> (6.7895, 2.0908)
  line L684 (6.7895, 2.0908) -> (6.7515, 1.9513)
  line L685 (6.7515, 1.9513) -> (6.7263, 1.8075)
  line L686 (6.7263, 1.8075) -> (6.7151, 1.6592)
  line L687 (6.7151, 1.6592) -> (6.7143, 1.5077)
  line L688 (6.7143, 1.5077) -> (6.7224, 1.3537)
  line L689 (6.7224, 1.3537) -> (6.7385, 1.1975)
  line L690 (6.7385, 1.1975) -> (6.7622, 1.0396)
  line L691 (6.7622, 1.0396) -> (6.7932, 0.8801)
  line L692 (6.7932, 0.8801) -> (6.8312, 0.7194)
  line L693 (6.8312, 0.7194) -> (6.8759, 0.5575)
  line L694 (6.8759, 0.5575) -> (6.9273, 0.3948)
  line L695 (6.9273, 0.3948) -> (6.9702, 0.2723)
  line L696 (6.9702, 0.2723) -> (7.5448, 0.1486)
  line L697 (7.5448, 0.1486) -> (7.6343, 0.2426)
  line L698 (7.6343, 0.2426) -> (7.7481, 0.3698)
  line L699 (7.7481, 0.3698) -> (7.8555, 0.4989)
  line L700 (7.8555, 0.4989) -> (7.9562, 0.6297)
  line L701 (7.9562, 0.6297) -> (8.0501, 0.7623)
  line L702 (8.0501, 0.7623) -> (8.1367, 0.8965)
  line L703 (8.1367, 0.8965) -> (8.2156, 1.0322)
  line L704 (8.2156, 1.0322) -> (8.2864, 1.1692)
  line L705 (8.2864, 1.1692) -> (8.348, 1.3076)
  line L706 (8.348, 1.3076) -> (8.3988, 1.4474)
  line L707 (8.3988, 1.4474) -> (8.4351, 1.5888)
  line L708 (8.4351, 1.5888) -> (8.4578, 1.7316)
  line L709 (8.4578, 1.7316) -> (8.4749, 1.8024)
  line L710 (8.4749, 1.8024) -> (8.4969, 1.8728)
  line L711 (8.4969, 1.8728) -> (8.5252, 1.9426)
  line L712 (8.5252, 1.9426) -> (8.5619, 2.0118)
  line L713 (8.5619, 2.0118) -> (8.5848, 2.046)
  line L714 (8.3803, 6.9208) -> (8.6977, 6.8314)
  line L715 (8.6977, 6.8314) -> (9.0243, 6.7862)
  line L716 (9.0243, 6.7862) -> (9.3539, 6.7859)
  line L717 (9.3539, 6.7859) -> (10.2051, 6.5218)
  line L718 (10.2051, 6.5218) -> (11.7219, 4.7363)
  line L719 (11.7219, 4.7363) -> (11.5995, 4.1427)
  line L720 (11.5995, 4.1427) -> (11.263, 3.9955)
  line L721 (11.263, 3.9955) -> (10.9176, 3.8707)
  line L722 (10.9176, 3.8707) -> (10.5647, 3.7689)
  line L723 (10.5647, 3.7689) -> (10.2059, 3.6904)
  line L724 (10.2059, 3.6904) -> (9.8427, 3.6357)
  line L725 (9.8427, 3.6357) -> (9.4767, 3.6049)
  line L726 (9.4767, 3.6049) -> (9.1094, 3.5981)
  line L727 (9.1094, 3.5981) -> (8.7426, 3.6156)
  line L728 (8.7426, 3.6156) -> (8.3776, 3.657)
  line L729 (8.3776, 3.657) -> (8.0162, 3.7223)
  line L730 (8.0162, 3.7223) -> (7.6598, 3.8112)
  line L731 (7.6598, 3.8112) -> (7.31, 3.9233)
  line L732 (7.31, 3.9233) -> (6.9684, 4.0581)
  line L733 (6.9684, 4.0581) -> (6.6363, 4.215)
  line L734 (6.6363, 4.215) -> (6.3152, 4.3934)
  line L735 (6.3152, 4.3934) -> (6.0066, 4.5925)
  line L736 (6.0066, 4.5925) -> (5.7116, 4.8114)
  line L737 (5.7116, 4.8114) -> (5.4317, 5.0492)
  line L738 (5.4317, 5.0492) -> (5.168, 5.3048)
  line L739 (5.168, 5.3048) -> (4.9216, 5.5772)
  line L740 (4.9216, 5.5772) -> (4.6936, 5.8652)
  line L741 (4.6936, 5.8652) -> (4.4851, 6.1676)
  line L742 (4.4851, 6.1676) -> (4.2968, 6.4829)
  line L743 (4.2968, 6.4829) -> (4.1296, 6.81)
  line L744 (4.1296, 6.81) -> (4.4109, 7.3469)
  line L745 (4.4109, 7.3469) -> (6.7155, 7.7678)
  line L746 (6.7155, 7.7678) -> (7.5415, 7.4331)
  line L747 (7.5415, 7.4331) -> (7.7968, 7.2245)
  line L748 (7.7968, 7.2245) -> (8.0781, 7.0526)
  line L749 (8.0781, 7.0526) -> (8.3803, 6.9208)
  line L750 (14.7474, 9.8325) -> (14.7775, 9.4665)
  line L751 (14.7775, 9.4665) -> (14.7836, 9.0993)
  line L752 (14.7836, 9.0993) -> (14.7655, 8.7324)
  line L753 (14.7655, 8.7324) -> (14.7234, 8.3675)
  line L754 (14.7234, 8.3675) -> (14.6574, 8.0062)
  line L755 (14.6574, 8.0062) -> (14.5679, 7.65)
  line L756 (14.5679, 7.65) -> (14.4551, 7.3004)
  line L757 (14.4551, 7.3004) -> (14.3197, 6.959)
  line L758 (14.3197, 6.959) -> (14.1622, 6.6272)
  line L759 (14.1622, 6.6272) -> (13.9832, 6.3065)
  line L760 (13.9832, 6.3065) -> (13.7836, 5.9982)
  line L761 (13.7836, 5.9982) -> (13.178, 5.9733)
  line L762 (13.178, 5.9733) -> (11.6611, 7.7587)
  line L763 (11.6611, 7.7587) -> (11.538, 8.6414)
  line L764 (11.538, 8.6414) -> (11.591, 8.9668)
  line L765 (11.591, 8.9668) -> (11.5992, 9.2964)
  line L766 (11.5992, 9.2964) -> (11.5623, 9.624)
  line L767 (11.5623, 9.624) -> (11.481, 9.9435)
  line L768 (11.481, 9.9435) -> (11.3569, 10.249)
  line L769 (11.3569, 10.249) -> (11.1922, 10.5346)
  line L770 (11.1922, 10.5346) -> (10.9954, 11.4038)
  line L771 (10.9954, 11.4038) -> (11.7832, 13.6101)
  line L772 (11.7832, 13.6101) -> (12.3585, 13.8009)
  line L773 (12.3585, 13.8009) -> (12.6543, 13.5831)
  line L774 (12.6543, 13.5831) -> (12.9351, 13.3463)
  line L775 (12.9351, 13.3463) -> (13.1997, 13.0917)
  line L776 (13.1997, 13.0917) -> (13.4471, 12.8202)
  line L777 (13.4471, 12.8202) -> (13.6761, 12.533)
  line L778 (13.6761, 12.533) -> (13.8857, 12.2314)
  line L779 (13.8857, 12.2314) -> (14.0752, 11.9168)
  line L780 (14.0752, 11.9168) -> (14.2435, 11.5903)
  line L781 (14.2435, 11.5903) -> (14.3901, 11.2535)
  line L782 (14.3901, 11.2535) -> (14.5143, 10.9079)
  line L783 (14.5143, 10.9079) -> (14.6155, 10.5548)
  line L784 (14.6155, 10.5548) -> (14.6933, 10.1958)
  line L785 (14.6933, 10.1958) -> (14.7474, 9.8325)
  circle A2 centre (9.1909, 9.1909) radius 0.5
  line L786 (9.2928, 14.7834) -> (9.6596, 14.7646)
  line L787 (9.6596, 14.7646) -> (9.9839, 14.2526)
  line L788 (9.9839, 14.2526) -> (9.1961, 12.0463)
  line L789 (9.1961, 12.0463) -> (8.4933, 11.4983)
  line L790 (8.4933, 11.4983) -> (8.185, 11.3816)
  line L791 (8.185, 11.3816) -> (7.8955, 11.2238)
  line L792 (7.8955, 11.2238) -> (7.6302, 11.028)
  line L793 (7.6302, 11.028) -> (7.3941, 10.7979)
  line L794 (7.3941, 10.7979) -> (7.1917, 10.5377)
  line L795 (7.1917, 10.5377) -> (7.0266, 10.2523)
  line L796 (7.0266, 10.2523) -> (6.3723, 9.6472)
  line L797 (6.3723, 9.6472) -> (4.0677, 9.2263)
  line L798 (4.0677, 9.2263) -> (3.6147, 9.6291)
  line L799 (3.6147, 9.6291) -> (3.6555, 9.9942)
  line L800 (3.6555, 9.9942) -> (3.7202, 10.3557)
  line L801 (3.7202, 10.3557) -> (3.8084, 10.7123)
  line L802 (3.8084, 10.7123) -> (3.9199, 11.0622)
  line L803 (3.9199, 11.0622) -> (4.0541, 11.4041)
  line L804 (4.0541, 11.4041) -> (4.2104, 11.7365)
  line L805 (4.2104, 11.7365) -> (4.3882, 12.0579)
  line L806 (4.3882, 12.0579) -> (4.5867, 12.3669)
  line L807 (4.5867, 12.3669) -> (4.8051, 12.6623)
  line L808 (4.8051, 12.6623) -> (5.0423, 12.9426)
  line L809 (5.0423, 12.9426) -> (5.2975, 13.2068)
  line L810 (5.2975, 13.2068) -> (5.5695, 13.4537)
  line L811 (5.5695, 13.4537) -> (5.857, 13.6822)
  line L812 (5.857, 13.6822) -> (6.159, 13.8913)
  line L813 (6.159, 13.8913) -> (6.474, 14.0801)
  line L814 (6.474, 14.0801) -> (6.8007, 14.2479)
  line L815 (6.8007, 14.2479) -> (7.1378, 14.3939)
  line L816 (7.1378, 14.3939) -> (7.4837, 14.5174)
  line L817 (7.4837, 14.5174) -> (7.837, 14.618)
  line L818 (7.837, 14.618) -> (8.196, 14.6951)
  line L819 (8.196, 14.6951) -> (8.5594, 14.7485)
  line L820 (8.5594, 14.7485) -> (8.9255, 14.778)
  line L821 (8.9255, 14.778) -> (9.2928, 14.7834)
  point P0 (0, 0)
  point P1 (9.1909, 9.1909)
  point P2 (8.5435, 9.953)
  point P3 (8.5879, 10.673)
  point P4 (7.8258, 10.0255)
  point P5 (8.8865, 7.6202)
  point P6 (10.7903, 9.2375)
  dimension "d2" = 3.2
  dimension "d3" = 2
  dimension "d6" = 1
  constraints: 20 end point, 7 midpoint, 4 parallel, 3 perpendicular, 2 coincident, 1 centre point, 1 tangent
  measures "d2" diameter of A0
  measures "d3" distance of L2.end L1.end
  measures "d6" distance of L7.end L8.end
extrude "Выдавливание2" cut sketch "Эскиз2" against normal through all contours L1 A0 L3 | L3 L7 A0 | A0 L9 L3 | L7 L3 L9 A0 | A0 L9 L794 L793 L792 L791 L7 | L791 L792 L6 L7 | L9 L6 L793 L794 | A1